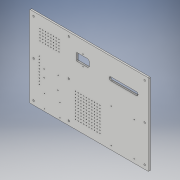
# Autodesk Inventor part: Electronics Base
Saved by Autodesk Inventor 2019 (Build 230136000, 136)
## iProperties
Created: 2020-07-20
Part Number: Electronics Base
Material: Generic
Document SubType Name: Modeling
Designer: Vijay
Density: 1 g/cm^3
Appearance: Default
Author: Vijay
Autodesk Inventor part; units mm, degrees
ref_plane "YZ Plane" through (0, 0, 0) normal (1, 0, 0) x (0, 1, 0)
ref_plane "XZ Plane" through (0, 0, 0) normal (0, 1, 0) x (-1, 0, 0)
ref_plane "XY Plane" through (0, 0, 0) normal (0, 0, 1) x (1, 0, 0)
sketch "Sketch1" plane through (0, 0, 0) normal (0, 0, 1) x (1, 0, 0)
  line L0 (28, 0) -> (28, -900) projected
  line L1 (-132, 0) -> (-132, -900) projected
  line L2 (-31.9999, 130.0003) -> (438.0001, 130.0005) projected
  line L3 (26, -170.1351) -> (-130, -170.1351)
  line L4 (-132, -168.1351) -> (-132, 127.8649)
  line L5 (-130, 129.8649) -> (26, 129.8649)
  line L6 (28, 127.8649) -> (28, -168.1351)
  arc A0 (26, -170.1351) -> (28, -168.1351) centre (26, -168.1351) ccw
  arc A1 (-132, -168.1351) -> (-130, -170.1351) centre (-130, -168.1351) ccw
  arc A2 (28, 127.8649) -> (26, 129.8649) centre (26, 127.8649) ccw
  arc A3 (-130, 129.8649) -> (-132, 127.8649) centre (-130, 127.8649) ccw
  point P0 (0, 0)
  point P1 (28, -170.1351)
  dimension "d0" = 300
  dimension "d1" = 2
  constraints: 8 end point, 8 point on circle, 8 tangent, 4 centre point, 3 equal radius, 3 point on line, 2 parallel, 1 horizontal, 1 perpendicular
  measures "d0" distance between parallel lines of L5 L3
  measures "d1" radius of A0
extrude "Extrusion1" add sketch "Sketch1" along normal blind 6
sketch "Sketch2" plane through (0, 0, 6) normal (0, 0, 1) x (1, 0, 0)
  line L0 (17.1, 100) -> (17.1, -900) construction
  line L1 (8.9, 100) -> (17.1, 100) construction
  line L2 (8.9, 100) -> (8.9, -900) construction
  line L3 (17.1, -900) -> (8.9, -900) construction
  line L4 (-112.9, 100) -> (-112.9, -900) construction
  line L5 (-121.1, 100) -> (-112.9, 100) construction
  line L6 (-121.1, 100) -> (-121.1, -900) construction
  line L7 (-112.9, -900) -> (-121.1, -900) construction
  line L8 (13, 100) -> (13, -217.6534) construction
  line L9 (-117, 100) -> (-117, -201.2401) construction
  line L10 (-131.9999, 119.1003) -> (438.0001, 119.1005) construction
  line L11 (-131.9999, 110.9003) -> (-131.9999, 119.1003) construction
  line L12 (-131.9999, 110.9003) -> (438.0001, 110.9005) construction
  line L13 (438.0001, 119.1005) -> (438.0001, 110.9005) construction
  line L14 (-132, 127.8649) -> (-132, -168.1351) construction
  line L15 (-132, 115.0005) -> (71.1699, 115.0005) construction
  circle A0 centre (13, 115.0005) radius 3
  circle A1 centre (-117, 115.0005) radius 3
  line L16 (28, -168.1351) -> (28, 127.8649) construction
  line L17 (28, -20.1351) -> (-209.5382, -20.1351) construction
  circle A2 centre (13, -20.1351) radius 3
  circle A3 centre (-117, -20.1351) radius 3
  circle A4 centre (13, -155.2707) radius 3
  circle A5 centre (-117, -155.2707) radius 3
  point P0 (0, 0)
  dimension "d4" = 6
  dimension "d5" = 6
  dimension "d6" = 6
  dimension "d7" = 6
  constraints: 8 end point, 7 point on line, 6 centre point, 3 midpoint, 3 parallel, 2 symmetric about line, 1 horizontal, 2 other
  measures "d4" diameter of A0
  measures "d5" diameter of A1
  measures "d6" diameter of A2
  measures "d7" diameter of A3
extrude "Extrusion2" cut sketch "Sketch2" against normal blind 10
sketch "Sketch3" plane through (0, 0, 6) normal (0, 0, 1) x (1, 0, 0)
  line L0 (309, 0) -> (309, 100) projected
  line L1 (26, 129.8649) -> (307, 129.8649)
  line L2 (309, 127.8649) -> (309, -168.1351)
  line L3 (307, -170.1351) -> (26, -170.1351)
  line L4 (26, -170.1351) -> (26, 129.8649)
  arc A0 (307, -170.1351) -> (309, -168.1351) centre (307, -168.1351) ccw
  arc A1 (309, 127.8649) -> (307, 129.8649) centre (307, 127.8649) ccw
  line L5 (298.1, 100) -> (298.1, -900) construction
  line L6 (289.9, 100) -> (298.1, 100) construction
  line L7 (289.9, 100) -> (289.9, -900) construction
  line L8 (298.1, -900) -> (289.9, -900) projected
  line L9 (294, 100) -> (294, -226.2133) construction
  circle A2 centre (13, 115.0005) radius 3 projected
  circle A3 centre (-117, 115.0005) radius 3 projected
  circle A4 centre (13, -155.2707) radius 3 projected
  circle A5 centre (-117, -155.2707) radius 3 projected
  circle A6 centre (13, -20.1351) radius 3 projected
  circle A7 centre (-117, -20.1351) radius 3 projected
  line L10 (-117, -155.2707) -> (365.5787, -155.2707) construction
  line L11 (-117, 115.0005) -> (393.0801, 115.0005) construction
  line L12 (-117, -20.1351) -> (365.5787, -20.1351) construction
  line L13 (294, 90.133) -> (294, 146.7932) construction
  circle A8 centre (294, -155.2707) radius 3
  circle A9 centre (294, -20.1351) radius 3
  circle A10 centre (294, 115.0005) radius 3
  point P0 (0, 0)
  point P1 (26, -170.1351)
  dimension "d10" = 2
  dimension "d11" = 6
  dimension "d12" = 6
  dimension "d13" = 6
  constraints: 18 end point, 7 point on line, 5 centre point, 4 horizontal, 4 point on circle, 4 tangent, 3 parallel, 1 equal radius, 1 midpoint, 1 perpendicular, 1 vertical
  measures "d10" radius of A0
  measures "d11" diameter of A8
  measures "d12" diameter of A9
  measures "d13" diameter of A10
extrude "Extrusion3" add sketch "Sketch3" against normal blind 6 contours L2 A0 L3 L4 L1 A1 L0
sketch "Sketch4" plane through (0, 0, 6) normal (0, 0, 1) x (1, 0, 0)
  circle A0 centre (-77.116, -161.7578) radius 1.3 projected
  circle A1 centre (-19.616, -161.7578) radius 1.3 projected
  circle A2 centre (-27.2256, -77.4445) radius 1.5875 projected
  circle A3 centre (-25.956, -29.2012) radius 1.5875 projected
  circle A4 centre (-78.026, -62.2212) radius 1.5875 projected
  circle A5 centre (-78.026, -34.2812) radius 1.5875 projected
  line L0 (73.7921, 78.7382) -> (43.8921, 78.7382) projected
  line L1 (73.7921, 53.7382) -> (73.7921, 78.7382) projected
  line L2 (61.8921, 53.7382) -> (73.7921, 53.7382) projected
  line L3 (61.8921, 51.2382) -> (61.8921, 53.7382) projected
  line L4 (43.8921, 51.2382) -> (61.8921, 51.2382) projected
  arc A6 (41.8921, 53.2382) -> (43.8921, 51.2382) centre (43.8921, 53.2382) ccw projected
  line L5 (41.8921, 76.7382) -> (41.8921, 53.2382) projected
  arc A7 (43.8921, 78.7382) -> (41.8921, 76.7382) centre (43.8921, 76.7382) ccw projected
  line L6 (42.8921, 53.4882) -> (42.8921, 76.4882) projected
  arc A8 (42.8921, 53.4882) -> (43.8921, 52.4882) centre (43.8921, 53.4882) ccw projected
  line L7 (57.8921, 52.4882) -> (43.8921, 52.4882) projected
  arc A9 (57.8921, 52.4882) -> (58.8921, 53.4882) centre (57.8921, 53.4882) ccw projected
  line L8 (58.8921, 76.4882) -> (58.8921, 53.4882) projected
  arc A10 (58.8921, 76.4882) -> (57.8921, 77.4882) centre (57.8921, 76.4882) ccw projected
  line L9 (43.8921, 77.4882) -> (57.8921, 77.4882) projected
  arc A11 (43.8921, 77.4882) -> (42.8921, 76.4882) centre (43.8921, 76.4882) ccw projected
  line L10 (83.3921, 78.7382) -> (80.3921, 78.7382) projected
  line L11 (83.3921, 78.7382) -> (89.8921, 72.2382) projected
  line L12 (89.8921, 57.7382) -> (89.8921, 72.2382) projected
  line L13 (89.8921, 57.7382) -> (83.3921, 51.2382) projected
  line L14 (80.3921, 51.2382) -> (83.3921, 51.2382) projected
  line L15 (80.3921, 78.7382) -> (80.3921, 51.2382) projected
  line L16 (80.3921, 51.2382) -> (61.8921, 51.2382)
  line L17 (80.3921, 78.7382) -> (73.7921, 78.7382)
  circle A12 centre (65.8921, 44.9882) radius 1.5 projected
  circle A13 centre (65.8921, 84.9882) radius 1.5 projected
  point P0 (0, 0)
  constraints: 4 end point, 2 parallel
extrude "Extrusion4" cut sketch "Sketch4" against normal blind 6 contours A0 | A1 | A2 | A3 | A4 | A5 | L1 L2 L3 L4 A6 L5 A7 L0 | L17 L15 L16 L3 L2 L1 | L10 L11 L12 L13 L14 L15 | L6 A11 L9 A10 L8 A9 L7 A8 | A12 | A13
sketch "Sketch5" plane through (0, 0, 0) normal (0, 0, -1) x (-1, 0, 0)
  circle A0 centre (78.026, -34.2812) radius 1.5875 projected
  circle A1 centre (25.956, -29.2012) radius 1.5875 projected
  circle A2 centre (-65.8921, 84.9882) radius 1.5 projected
  circle A3 centre (19.616, -161.7578) radius 1.3 projected
  circle A4 centre (77.116, -161.7578) radius 1.3 projected
  circle A5 centre (-65.8921, 44.9882) radius 1.5 projected
  circle A6 centre (27.2256, -77.4445) radius 1.5875 projected
  circle A7 centre (78.026, -62.2212) radius 1.5875 projected
  line L0 (-83.3921, 51.2382) -> (-89.8921, 57.7382) projected
  line L1 (-89.8921, 57.7382) -> (-89.8921, 72.2382) projected
  line L2 (-89.8921, 72.2382) -> (-83.3921, 78.7382) projected
  line L3 (-83.3921, 78.7382) -> (-43.8921, 78.7382) projected
  arc A8 (-41.8921, 76.7382) -> (-43.8921, 78.7382) centre (-43.8921, 76.7382) ccw projected
  line L4 (-41.8921, 76.7382) -> (-41.8921, 53.2382) projected
  arc A9 (-43.8921, 51.2382) -> (-41.8921, 53.2382) centre (-43.8921, 53.2382) ccw projected
  line L5 (-43.8921, 51.2382) -> (-83.3921, 51.2382) projected
  line L6 (130, -170.1351) -> (-307, -170.1351) projected
  arc A10 (130, -170.1351) -> (132, -168.1351) centre (130, -168.1351) ccw projected
  line L7 (132, 127.8649) -> (132, -168.1351) projected
  arc A11 (132, 127.8649) -> (130, 129.8649) centre (130, 127.8649) ccw projected
  line L8 (130, 129.8649) -> (-307, 129.8649) projected
  arc A12 (-307, 129.8649) -> (-309, 127.8649) centre (-307, 127.8649) ccw projected
  line L9 (-309, 127.8649) -> (-309, -168.1351) projected
  arc A13 (-309, -168.1351) -> (-307, -170.1351) centre (-307, -168.1351) ccw projected
  circle A14 centre (-294, 115.0005) radius 3 projected
  circle A15 centre (-294, -20.1351) radius 3 projected
  circle A16 centre (-294, -155.2707) radius 3 projected
  circle A17 centre (-13, -155.2707) radius 3 projected
  circle A18 centre (-13, -20.1351) radius 3 projected
  circle A19 centre (-13, 115.0005) radius 3 projected
  circle A20 centre (117, 115.0005) radius 3 projected
  circle A21 centre (117, -20.1351) radius 3 projected
  circle A22 centre (117, -155.2707) radius 3 projected
  line L10 (-83.475, 51.0382) -> (-90.0921, 57.6554)
  line L11 (-90.0921, 57.6554) -> (-90.0921, 72.321)
  line L12 (-90.0921, 72.321) -> (-83.475, 78.9382)
  line L13 (-83.475, 78.9382) -> (-43.8921, 78.9382)
  arc A23 (-41.6921, 76.7382) -> (-43.8921, 78.9382) centre (-43.8921, 76.7382) ccw
  line L14 (-41.6921, 76.7382) -> (-41.6921, 53.2382)
  arc A24 (-43.8921, 51.0382) -> (-41.6921, 53.2382) centre (-43.8921, 53.2382) ccw
  line L15 (-43.8921, 51.0382) -> (-83.475, 51.0382)
  point P0 (0, 0)
  dimension "d18" = 0.2
  constraints: 12 end point, 4 point on circle, 2 centre point, 7 other
  measures "d18" distance between parallel lines of L5 L15
extrude "Extrusion5" cut sketch "Sketch5" against normal blind 6 contours L10 L11 L12 L13 A23 L14 A24 L15
sketch "Sketch6" plane through (0, 0, 6) normal (0, 0, 1) x (1, 0, 0)
  circle A0 centre (255.3223, -29.828) radius 1.5 projected
  circle A1 centre (170.3223, -29.828) radius 1.5 projected
  circle A2 centre (170.3223, -155.828) radius 1.5 projected
  circle A3 centre (255.3223, -155.828) radius 1.5 projected
  point P0 (0, 0)
extrude "Extrusion6" cut sketch "Sketch6" against normal blind 6
sketch "Sketch7" plane through (0, 0, 6) normal (0, 0, 1) x (1, 0, 0)
  line L0 (263.156, 57.3706) -> (168.9988, 57.3706) construction
  line L1 (263.156, 63.8271) -> (168.9988, 63.8271)
  line L2 (168.9988, 50.9141) -> (263.156, 50.9141)
  arc A0 (263.156, 50.9141) -> (263.156, 63.8271) centre (263.156, 57.3706) ccw
  arc A1 (168.9988, 63.8271) -> (168.9988, 50.9141) centre (168.9988, 57.3706) ccw
  point P0 (0, 0)
  point P1 (216.0774, 57.3706)
  constraints: 8 end point, 4 point on circle, 4 tangent, 2 centre point, 1 horizontal, 1 midpoint, 1 parallel
extrude "Extrusion7" cut sketch "Sketch7" against normal blind 6
sketch "Sketch8" plane through (0, 0, 6) normal (0, 0, 1) x (1, 0, 0)
  circle A0 centre (128.1075, -138.0817) radius 1.5
  line L0 (-130, -170.1351) -> (307, -170.1351) projected
  line L1 (-132, 127.8649) -> (-132, -168.1351) projected
  circle A1 centre (118.1075, -138.0817) radius 1.5
  circle A2 centre (108.1075, -138.0817) radius 1.5
  circle A3 centre (98.1075, -138.0817) radius 1.5
  circle A4 centre (88.1075, -138.0817) radius 1.5
  circle A5 centre (78.1075, -138.0817) radius 1.5
  circle A6 centre (68.1075, -138.0817) radius 1.5
  circle A7 centre (58.1075, -138.0817) radius 1.5
  circle A8 centre (48.1075, -138.0817) radius 1.5
  circle A9 centre (38.1075, -138.0817) radius 1.5
  circle A10 centre (128.1075, -128.0817) radius 1.5
  circle A11 centre (118.1075, -128.0817) radius 1.5
  circle A12 centre (108.1075, -128.0817) radius 1.5
  circle A13 centre (98.1075, -128.0817) radius 1.5
  circle A14 centre (88.1075, -128.0817) radius 1.5
  circle A15 centre (78.1075, -128.0817) radius 1.5
  circle A16 centre (68.1075, -128.0817) radius 1.5
  circle A17 centre (58.1075, -128.0817) radius 1.5
  circle A18 centre (48.1075, -128.0817) radius 1.5
  circle A19 centre (38.1075, -128.0817) radius 1.5
  circle A20 centre (128.1075, -118.0817) radius 1.5
  circle A21 centre (118.1075, -118.0817) radius 1.5
  circle A22 centre (108.1075, -118.0817) radius 1.5
  circle A23 centre (98.1075, -118.0817) radius 1.5
  circle A24 centre (88.1075, -118.0817) radius 1.5
  circle A25 centre (78.1075, -118.0817) radius 1.5
  circle A26 centre (68.1075, -118.0817) radius 1.5
  circle A27 centre (58.1075, -118.0817) radius 1.5
  circle A28 centre (48.1075, -118.0817) radius 1.5
  circle A29 centre (38.1075, -118.0817) radius 1.5
  circle A30 centre (128.1075, -108.0817) radius 1.5
  circle A31 centre (118.1075, -108.0817) radius 1.5
  circle A32 centre (108.1075, -108.0817) radius 1.5
  circle A33 centre (98.1075, -108.0817) radius 1.5
  circle A34 centre (88.1075, -108.0817) radius 1.5
  circle A35 centre (78.1075, -108.0817) radius 1.5
  circle A36 centre (68.1075, -108.0817) radius 1.5
  circle A37 centre (58.1075, -108.0817) radius 1.5
  circle A38 centre (48.1075, -108.0817) radius 1.5
  circle A39 centre (38.1075, -108.0817) radius 1.5
  circle A40 centre (128.1075, -98.0817) radius 1.5
  circle A41 centre (118.1075, -98.0817) radius 1.5
  circle A42 centre (108.1075, -98.0817) radius 1.5
  circle A43 centre (98.1075, -98.0817) radius 1.5
  circle A44 centre (88.1075, -98.0817) radius 1.5
  circle A45 centre (78.1075, -98.0817) radius 1.5
  circle A46 centre (68.1075, -98.0817) radius 1.5
  circle A47 centre (58.1075, -98.0817) radius 1.5
  circle A48 centre (48.1075, -98.0817) radius 1.5
  circle A49 centre (38.1075, -98.0817) radius 1.5
  circle A50 centre (128.1075, -88.0817) radius 1.5
  circle A51 centre (118.1075, -88.0817) radius 1.5
  circle A52 centre (108.1075, -88.0817) radius 1.5
  circle A53 centre (98.1075, -88.0817) radius 1.5
  circle A54 centre (88.1075, -88.0817) radius 1.5
  circle A55 centre (78.1075, -88.0817) radius 1.5
  circle A56 centre (68.1075, -88.0817) radius 1.5
  circle A57 centre (58.1075, -88.0817) radius 1.5
  circle A58 centre (48.1075, -88.0817) radius 1.5
  circle A59 centre (38.1075, -88.0817) radius 1.5
  circle A60 centre (128.1075, -78.0817) radius 1.5
  circle A61 centre (118.1075, -78.0817) radius 1.5
  circle A62 centre (108.1075, -78.0817) radius 1.5
  circle A63 centre (98.1075, -78.0817) radius 1.5
  circle A64 centre (88.1075, -78.0817) radius 1.5
  circle A65 centre (78.1075, -78.0817) radius 1.5
  circle A66 centre (68.1075, -78.0817) radius 1.5
  circle A67 centre (58.1075, -78.0817) radius 1.5
  circle A68 centre (48.1075, -78.0817) radius 1.5
  circle A69 centre (38.1075, -78.0817) radius 1.5
  circle A70 centre (128.1075, -68.0817) radius 1.5
  circle A71 centre (118.1075, -68.0817) radius 1.5
  circle A72 centre (108.1075, -68.0817) radius 1.5
  circle A73 centre (98.1075, -68.0817) radius 1.5
  circle A74 centre (88.1075, -68.0817) radius 1.5
  circle A75 centre (78.1075, -68.0817) radius 1.5
  circle A76 centre (68.1075, -68.0817) radius 1.5
  circle A77 centre (58.1075, -68.0817) radius 1.5
  circle A78 centre (48.1075, -68.0817) radius 1.5
  circle A79 centre (38.1075, -68.0817) radius 1.5
  circle A80 centre (128.1075, -58.0817) radius 1.5
  circle A81 centre (118.1075, -58.0817) radius 1.5
  circle A82 centre (108.1075, -58.0817) radius 1.5
  circle A83 centre (98.1075, -58.0817) radius 1.5
  circle A84 centre (88.1075, -58.0817) radius 1.5
  circle A85 centre (78.1075, -58.0817) radius 1.5
  circle A86 centre (68.1075, -58.0817) radius 1.5
  circle A87 centre (58.1075, -58.0817) radius 1.5
  circle A88 centre (48.1075, -58.0817) radius 1.5
  circle A89 centre (38.1075, -58.0817) radius 1.5
  circle A90 centre (128.1075, -48.0817) radius 1.5
  circle A91 centre (118.1075, -48.0817) radius 1.5
  circle A92 centre (108.1075, -48.0817) radius 1.5
  circle A93 centre (98.1075, -48.0817) radius 1.5
  circle A94 centre (88.1075, -48.0817) radius 1.5
  circle A95 centre (78.1075, -48.0817) radius 1.5
  circle A96 centre (68.1075, -48.0817) radius 1.5
  circle A97 centre (58.1075, -48.0817) radius 1.5
  circle A98 centre (48.1075, -48.0817) radius 1.5
  circle A99 centre (38.1075, -48.0817) radius 1.5
  circle A100 centre (-95.9152, -92.7899) radius 1.5
  circle A101 centre (-95.9152, -82.7899) radius 1.5
  circle A102 centre (-95.9152, -72.7899) radius 1.5
  circle A103 centre (-95.9152, -62.7899) radius 1.5
  circle A104 centre (-95.9152, -52.7899) radius 1.5
  circle A105 centre (-95.9152, -42.7899) radius 1.5
  circle A106 centre (-95.9152, -32.7899) radius 1.5
  circle A107 centre (-95.9152, -22.7899) radius 1.5
  circle A108 centre (-95.9152, -12.7899) radius 1.5
  circle A109 centre (-95.9152, -2.7899) radius 1.5
  point P0 (0, 0)
  dimension "d25" = 3
  dimension "d28" = 10
  dimension "d31" = 10
  dimension "d34" = 3
  dimension "d37" = 10
  constraints: 110 centre point, 2 vertical, 1 horizontal, 216 other
  measures "d25" diameter of A0
  measures "d28" distance of A0.centre A1.centre
  measures "d31" distance of A0.centre A10.centre
  measures "d34" diameter of A100
  measures "d37" distance of A100.centre A101.centre
extrude "Extrusion8" cut sketch "Sketch8" against normal blind 6
sketch "Sketch9" plane through (0, 0, 6) normal (0, 0, 1) x (1, 0, 0)
  circle A0 centre (-23.407, 47.4245) radius 1.5
  line L0 (-130, -170.1351) -> (307, -170.1351) projected
  line L1 (-132, 127.8649) -> (-132, -168.1351) projected
  circle A1 centre (-33.407, 47.4245) radius 1.5
  circle A2 centre (-43.407, 47.4245) radius 1.5
  circle A3 centre (-53.407, 47.4245) radius 1.5
  circle A4 centre (-63.407, 47.4245) radius 1.5
  circle A5 centre (-73.407, 47.4245) radius 1.5
  circle A6 centre (-83.407, 47.4245) radius 1.5
  circle A7 centre (-93.407, 47.4245) radius 1.5
  circle A8 centre (-23.407, 57.4245) radius 1.5
  circle A9 centre (-33.407, 57.4245) radius 1.5
  circle A10 centre (-43.407, 57.4245) radius 1.5
  circle A11 centre (-53.407, 57.4245) radius 1.5
  circle A12 centre (-63.407, 57.4245) radius 1.5
  circle A13 centre (-73.407, 57.4245) radius 1.5
  circle A14 centre (-83.407, 57.4245) radius 1.5
  circle A15 centre (-93.407, 57.4245) radius 1.5
  circle A16 centre (-23.407, 67.4245) radius 1.5
  circle A17 centre (-33.407, 67.4245) radius 1.5
  circle A18 centre (-43.407, 67.4245) radius 1.5
  circle A19 centre (-53.407, 67.4245) radius 1.5
  circle A20 centre (-63.407, 67.4245) radius 1.5
  circle A21 centre (-73.407, 67.4245) radius 1.5
  circle A22 centre (-83.407, 67.4245) radius 1.5
  circle A23 centre (-93.407, 67.4245) radius 1.5
  circle A24 centre (-23.407, 77.4245) radius 1.5
  circle A25 centre (-33.407, 77.4245) radius 1.5
  circle A26 centre (-43.407, 77.4245) radius 1.5
  circle A27 centre (-53.407, 77.4245) radius 1.5
  circle A28 centre (-63.407, 77.4245) radius 1.5
  circle A29 centre (-73.407, 77.4245) radius 1.5
  circle A30 centre (-83.407, 77.4245) radius 1.5
  circle A31 centre (-93.407, 77.4245) radius 1.5
  circle A32 centre (-23.407, 87.4245) radius 1.5
  circle A33 centre (-33.407, 87.4245) radius 1.5
  circle A34 centre (-43.407, 87.4245) radius 1.5
  circle A35 centre (-53.407, 87.4245) radius 1.5
  circle A36 centre (-63.407, 87.4245) radius 1.5
  circle A37 centre (-73.407, 87.4245) radius 1.5
  circle A38 centre (-83.407, 87.4245) radius 1.5
  circle A39 centre (-93.407, 87.4245) radius 1.5
  point P0 (0, 0)
  dimension "d44" = 3
  dimension "d47" = 10
  dimension "d50" = 10
  constraints: 40 centre point, 1 horizontal, 1 vertical, 78 other
  measures "d44" diameter of A0
  measures "d47" distance of A0.centre A1.centre
  measures "d50" distance of A0.centre A8.centre
extrude "Extrusion9" cut sketch "Sketch9" against normal blind 6
sketch "Sketch10" plane through (0, 0, 6) normal (0, 0, 1) x (1, 0, 0)
  circle A0 centre (-19.616, -112.6578) radius 1.3 projected
  circle A1 centre (-77.116, -112.6578) radius 1.3 projected
  point P0 (0, 0)
extrude "Extrusion10" cut sketch "Sketch10" against normal blind 6
body "Solid1"
